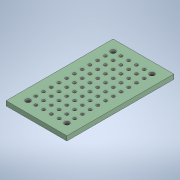
# Autodesk Inventor part: PCB_PowerSupply
Saved by Autodesk Inventor 2021 (Build 250183000, 183)
## iProperties
Created: 2021-08-02
Part Number: PCB_PowerSupply
Material: Generisch
Document SubType Name: Modeling
Designer: User
Density: 1 g/cm^3
Appearance: Vorgabe
Author: User
Autodesk Inventor part; units mm, degrees
ref_plane "YZ Plane" through (0, 0, 0) normal (1, 0, 0) x (0, 1, 0)
ref_plane "XZ Plane" through (0, 0, 0) normal (0, 1, 0) x (-1, 0, 0)
ref_plane "XY Plane" through (0, 0, 0) normal (0, 0, 1) x (1, 0, 0)
sketch "Skizze1" plane through (0, 0, 0) normal (0, 1, 0) x (-1, 0, 0)
  line L0 (10, 17.6) -> (-10, 17.6)
  line L1 (-10, 17.6) -> (-10, -17.6)
  line L2 (-10, -17.6) -> (10, -17.6)
  line L3 (10, -17.6) -> (10, 17.6)
  line L4 (6.4, 14) -> (-6.4, 14) construction
  line L5 (-6.4, 14) -> (-6.4, -14) construction
  line L6 (-6.4, -14) -> (6.4, -14) construction
  line L7 (6.4, -14) -> (6.4, 14) construction
  line L8 (0, 17.6) -> (0, -17.6) construction
  line L9 (10, 0) -> (-10, 0) construction
  point P0 (0, 0)
  point P1 (0, 0)
  dimension "d0" = 12.8
  dimension "d1" = 28
  dimension "d2" = 20
  dimension "d3" = 3.6
  dimension "d4" = 3.6
  constraints: 20 end point, 5 midpoint, 4 parallel, 2 coincident, 2 horizontal, 2 perpendicular, 2 other
  measures "d0" distance of L5.end L6.end
  measures "d1" distance of L4.end L5.end
  measures "d2" distance of L1.end L2.end
  measures "d3" distance between parallel lines of L3 L7
  measures "d4" distance between parallel lines of L2 L6
extrude "Extrusion1" add sketch "Skizze1" along normal blind 1.5
hole "Bohrung1" at (6.4, 0, 14) direction (0, 1, 0) diameter 1 end through all
pattern_linear "Rechteckige Anordnung1" count 12 spacing 2.5455 along (0, 0, -1) count 6 spacing 2.56 along (-1, 0, 0) of "Bohrung1"
sketch "Skizze2" plane through (0, 0, 0) normal (0, -1, 0) x (1, 0, 0)
  circle A0 centre (6.4, 14) radius 0.5 projected
  circle A1 centre (-6.4, 14) radius 0.5 projected
  circle A2 centre (-6.4, -14) radius 0.5 projected
  circle A3 centre (6.4, -14) radius 0.5 projected
  circle A4 centre (-6.4, -14) radius 0.5 projected
  point P0 (0, 0)
  constraints: 4 coincident
hole "Bohrung2" at (6.4, 0, -14) at (-6.4, 0, -14) at (-6.4, 0, 14) at (6.4, 0, 14) direction (0, 1, 0) diameter 1.6 end through all
equation "\"d4\" = d3"
